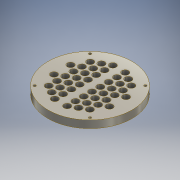
# Autodesk Inventor part: Tube Sheet
Saved by Autodesk Inventor 2016 (Build 200138000, 138)
## iProperties
Created: 2018-11-09
Part Number: Tube Sheet
Material: Titanium
Document SubType Name: Modeling
Designer: Wijaya
Density: 4.51 g/cm^3
Appearance: Titanium - Polished
Mass: 7468.29 g
Surface Area: 2531.27 cm^2
Volume: 1655.94 cm^3
Author: Wijaya
Autodesk Inventor part; units mm, degrees
note: some values were not read from the file. Chosen so that the rebuilt part matches the saved one: direction of "Hole2"; direction of "Hole3".
ref_plane "YZ Plane" through (0, 0, 0) normal (1, 0, 0) x (0, 1, 0)
ref_plane "XZ Plane" through (0, 0, 0) normal (0, 1, 0) x (-1, 0, 0)
ref_plane "XY Plane" through (0, 0, 0) normal (0, 0, 1) x (1, 0, 0)
sketch "Sketch1" plane through (0, 0, 0) normal (0, 0, 1) x (1, 0, 0)
  circle A0 centre (0, 0) radius 161.1083
  line L0 (4.75, 161.0382) -> (4.75, -161.0382)
  line L1 (-4.75, -161.0382) -> (-4.75, 161.0382)
  line L2 (0, 0) -> (0, 161.1083) construction
  line L3 (23.8125, 79.375) -> (23.8125, 47.625)
  line L4 (23.8125, 47.625) -> (51.3088, 63.5)
  line L5 (51.3088, 63.5) -> (23.8125, 79.375)
  line L6 (23.8125, 111.125) -> (23.8125, 79.375)
  line L7 (23.8125, 79.375) -> (51.3088, 95.25)
  line L8 (51.3088, 95.25) -> (23.8125, 111.125)
  line L9 (23.8125, 47.625) -> (23.8125, 15.875)
  line L10 (23.8125, 15.875) -> (51.3088, 31.75)
  line L11 (51.3088, 31.75) -> (23.8125, 47.625)
  line L12 (23.8125, 15.875) -> (23.8125, -15.875)
  line L13 (23.8125, -15.875) -> (51.3088, 0)
  line L14 (51.3088, 0) -> (23.8125, 15.875)
  line L15 (23.8125, -15.875) -> (23.8125, -47.625)
  line L16 (23.8125, -47.625) -> (51.3088, -31.75)
  line L17 (51.3088, -31.75) -> (23.8125, -15.875)
  line L18 (23.8125, -47.625) -> (23.8125, -79.375)
  line L19 (23.8125, -79.375) -> (51.3088, -63.5)
  line L20 (51.3088, -63.5) -> (23.8125, -47.625)
  line L21 (23.8125, -79.375) -> (23.8125, -111.125)
  line L22 (23.8125, -111.125) -> (51.3088, -95.25)
  line L23 (51.3088, -95.25) -> (23.8125, -79.375)
  line L24 (51.3088, 95.25) -> (78.8051, 79.375)
  line L25 (78.8051, 79.375) -> (51.3088, 63.5)
  line L26 (51.3088, 63.5) -> (78.8051, 47.625)
  line L27 (78.8051, 47.625) -> (51.3088, 31.75)
  line L28 (51.3088, 31.75) -> (78.8051, 15.875)
  line L29 (78.8051, 15.875) -> (51.3088, 0)
  line L30 (51.3088, 0) -> (78.8051, -15.875)
  line L31 (78.8051, -15.875) -> (51.3088, -31.75)
  line L32 (51.3088, -31.75) -> (78.8051, -47.625)
  line L33 (78.8051, -47.625) -> (51.3088, -63.5)
  line L34 (51.3088, -63.5) -> (78.8051, -79.375)
  line L35 (78.8051, -79.375) -> (51.3088, -95.25)
  line L36 (78.8051, -47.625) -> (106.3014, -31.75)
  line L37 (106.3014, -31.75) -> (78.8051, -15.875)
  line L38 (78.8051, -15.875) -> (106.3014, 0)
  line L39 (106.3014, 0) -> (78.8051, 15.875)
  line L40 (78.8051, 15.875) -> (106.3014, 31.75)
  line L41 (106.3014, 31.75) -> (78.8051, 47.625)
  line L42 (0, 0) -> (106.066, 106.066) construction
  point P0 (23.8125, 0)
  point P1 (78.8051, 79.375)
  dimension "d0" = 322.2165
  dimension "d2" = 9.5
  dimension "d3" = 4.75
  dimension "d4" = 31.75
  dimension "d5" = 31.75
  dimension "d6" = 31.75
  dimension "d7" = 31.75
  dimension "d8" = 31.75
  dimension "d9" = 31.75
  dimension "d10" = 31.75
  dimension "d27" = 23.8125
  dimension "d28" = 150
  dimension "d29" = 45
  constraints: 86 end point, 25 equal length, 9 coincident, 8 vertical, 7 parallel, 6 point on line, 4 point on circle, 1 centre point, 1 collinear, 1 horizontal alignment, 1 midpoint
  measures "d0" diameter of A0
  measures "d2" distance between parallel lines of L0 L1
  measures "d3" distance from line of L1 point (0, 0)
  measures "d4" distance of L3.start L4.end
  measures "d5" distance of L7.end L6.start
  measures "d6" distance of L3.end L10.end
  measures "d7" distance of L13.end L9.end
  measures "d8" distance of L12.end L16.end
  measures "d9" distance of L15.end L19.end
  measures "d10" distance of L18.end L22.end
  measures "d27" distance of point (0, 0) point (23.813, 0)
  measures "d28" distance of L2.start L42.end
  measures "d29" angle of L2 L42
extrude "Extrusion1" add sketch "Sketch1" along normal blind 28.575 contours A0 L0 | L0 A0 L1 | L1 A0 | L5 L4 L3 | L7 L24 L25 L5 | L6 L8 L7 | L11 L10 L9 | L4 L26 L27 L11 | L14 L13 L12 | L10 L28 L29 L14 | L27 L41 L40 L28 | L17 L16 L15 | L13 L30 L31 L17 | L29 L39 L38 L30 | L20 L19 L18 | L16 L32 L33 L20 | L31 L37 L36 L32 | L23 L22 L21 | L19 L34 L35 L23
hole "Hole2" at (23.8125, 47.625, 0) at (51.3088, 63.5, 0) at (23.8125, 111.125, 0) at (23.8125, 79.375, 0) at (51.3088, 95.25, 0) at (51.3088, 31.75, 0) at (23.8125, 15.875, 0) at (23.8125, -15.875, 0) at (51.3088, 0, 0) at (23.8125, -47.625, 0) at (51.3088, -31.75, 0) at (23.8125, -79.375, 0) at (51.3088, -63.5, 0) at (23.8125, -111.125, 0) at (51.3088, -95.25, 0) at (78.8051, 79.375, 0) at (78.8051, 47.625, 0) at (78.8051, 15.875, 0) at (78.8051, -15.875, 0) at (78.8051, -47.625, 0) at (78.8051, -79.375, 0) at (106.3014, -31.75, 0) at (106.3014, 31.75, 0) direction (0, 0, 1) diameter 25.4 end up to surface
mirror "Mirror1" about plane through (0, 0, 0) normal (1, 0, 0) of "Hole2"
hole "Hole3" at (106.066, 106.066, 0) direction (0, 0, 1) diameter 9.5 end up to surface
pattern_circular "Circular Pattern1" count 4 over 360 about axis through (0, 0, 0) along (0, 0, 1) of "Hole3"
body "Solid1"
